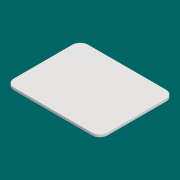
# Autodesk Inventor part: Boden
Saved by Autodesk Inventor 2020.1 (Build 241239000, 239)
## iProperties
Created: 2020-01-27
Part Number: Boden
Material: Generic
Document SubType Name: Modeling
Designer: Pluscrafter
Density: 1 g/cm^3
Appearance: Default
Author: Pluscrafter
Autodesk Inventor part; units mm, degrees
ref_plane "YZ Plane" through (0, 0, 0) normal (1, 0, 0) x (0, 1, 0)
ref_plane "XZ Plane" through (0, 0, 0) normal (0, 1, 0) x (-1, 0, 0)
ref_plane "XY Plane" through (0, 0, 0) normal (0, 0, 1) x (1, 0, 0)
sketch "Sketch1" plane through (0, 0, 0) normal (0, 1, 0) x (-1, 0, 0)
  line L0 (45.8955, 52.7129) -> (-54.1045, 52.7129)
  line L1 (-64.1045, 42.7129) -> (-64.1045, -32.2871)
  line L2 (-54.1045, -42.2871) -> (45.8955, -42.2871)
  line L3 (55.8955, -32.2871) -> (55.8955, 42.7129)
  arc A0 (-64.1045, -32.2871) -> (-54.1045, -42.2871) centre (-54.1045, -32.2871) ccw
  arc A1 (-54.1045, 52.7129) -> (-64.1045, 42.7129) centre (-54.1045, 42.7129) ccw
  arc A2 (55.8955, 42.7129) -> (45.8955, 52.7129) centre (45.8955, 42.7129) ccw
  arc A3 (45.8955, -42.2871) -> (55.8955, -32.2871) centre (45.8955, -32.2871) ccw
  point P0 (0, 0)
  dimension "d0" = 120
  dimension "d1" = 95
  dimension "d4" = 10
  constraints: 8 end point, 8 point on circle, 8 tangent, 4 centre point, 3 equal radius, 2 parallel, 1 horizontal, 1 perpendicular
  measures "d0" distance between parallel lines of L1 L3
  measures "d1" distance between parallel lines of L0 L2
  measures "d4" radius of A0
extrude "Extrusion2" add sketch "Sketch1" along normal blind 3
sketch "Sketch3" plane through (0, 3, 0) normal (0, 1, 0) x (1, 0, 0)
  line L0 (-40.8955, -28.7129) -> (-8.6955, -28.7129)
  line L1 (-8.6955, -28.7129) -> (-8.6955, -25.7129)
  line L2 (-8.6955, -25.7129) -> (-40.8955, -25.7129)
  line L3 (-40.8955, -25.7129) -> (-40.8955, -28.7129)
  line L4 (-40.8955, 15.2871) -> (-8.6955, 15.2871)
  line L5 (-8.6955, 15.2871) -> (-8.6955, 18.2871)
  line L6 (-8.6955, 18.2871) -> (-40.8955, 18.2871)
  line L7 (-40.8955, 18.2871) -> (-40.8955, 15.2871)
  line L8 (-29.7955, -28.7129) -> (-19.7955, -28.7129)
  line L9 (-19.7955, -28.7129) -> (-19.7955, -25.7129)
  line L10 (-19.7955, -25.7129) -> (-29.7955, -25.7129)
  line L11 (-29.7955, -25.7129) -> (-29.7955, -28.7129)
  line L12 (-29.7955, 15.2871) -> (-19.7955, 15.2871)
  line L13 (-19.7955, 15.2871) -> (-19.7955, 18.2871)
  line L14 (-19.7955, 18.2871) -> (-29.7955, 18.2871)
  line L15 (-29.7955, 18.2871) -> (-29.7955, 15.2871)
  line L16 (-55.8955, 32.2871) -> (-55.8955, -42.7129) projected
  line L17 (-45.8955, -52.7129) -> (54.1045, -52.7129) projected
  line L18 (54.1045, 42.2871) -> (-45.8955, 42.2871) projected
  point P0 (0, 0)
  point P1 (-8.6955, -27.2129)
  point P2 (-8.6955, 16.7871)
  dimension "d7" = 32.2
  dimension "d8" = 3
  dimension "d9" = 32.2
  dimension "d10" = 3
  dimension "d11" = 41
  dimension "d12" = 10
  dimension "d13" = 11.1
  dimension "d14" = 10
  dimension "d15" = 11.1
  dimension "d16" = 15
  dimension "d17" = 24
  dimension "d18" = 95
  dimension "d19" = 24
  constraints: 32 end point, 8 parallel, 4 horizontal, 4 perpendicular, 4 point on line, 2 midpoint, 1 vertical alignment
  measures "d7" distance of L2.end L1.end
  measures "d8" distance between parallel lines of L2 L0
  measures "d9" distance of L6.end L5.end
  measures "d10" distance between parallel lines of L6 L4
  measures "d11" distance between parallel lines of L4 L2
  measures "d12" distance of L10.end L9.end
  measures "d13" distance between parallel lines of L3 L11
  measures "d14" distance of L14.end L13.end
  measures "d15" distance between parallel lines of L15 L7
  measures "d16" distance between parallel lines of L16 L3
  measures "d17" distance between parallel lines of L17 L0
  measures "d18" distance between parallel lines of L18 L17
  measures "d19" distance between parallel lines of L18 L6
extrude "Extrusion3" cut sketch "Sketch3" against normal blind 10 contours L3 L2 L11 L0 | L9 L2 L1 L0 | L7 L6 L15 L4 | L13 L6 L5 L4
body "Solid2"
